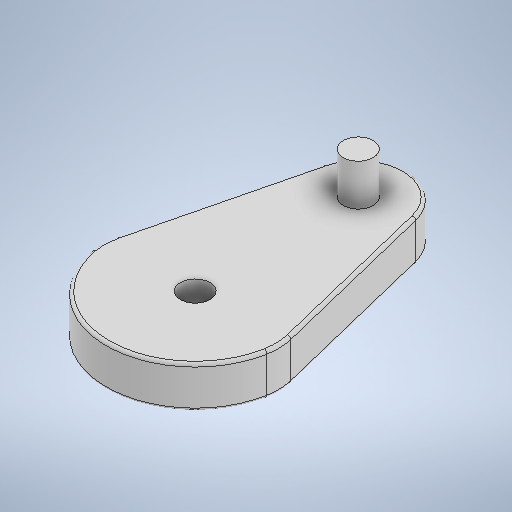
# Autodesk Inventor part: 202 part 1
Saved by Autodesk Inventor 2025.1 (Build 291241000, 241)
## iProperties
Created: 2024-09-02
Part Number: 202 part 1
Material: Generisch
Document SubType Name: Modeling
Designer: ffogue
Density: 1 g/cm^3
Appearance: Vorgabe
Author: ffogue
Autodesk Inventor part; units mm, degrees
ref_plane "YZ Plane" through (0, 0, 0) normal (1, 0, 0) x (0, 1, 0)
ref_plane "XZ Plane" through (0, 0, 0) normal (0, 1, 0) x (-1, 0, 0)
ref_plane "XY Plane" through (0, 0, 0) normal (0, 0, 1) x (1, 0, 0)
sketch "Sketch1" plane through (0, 0, 0) normal (0, 0, 1) x (1, 0, 0)
  line L0 (-15, 0) -> (15, 0) construction
  arc A0 (-15, 0) -> (15, 0) centre (0, 0) ccw
  line L1 (-15, 0) -> (-7.7686, 29.4102)
  arc A1 (7.7686, 29.4102) -> (-7.7686, 29.4102) centre (0, 27.5) ccw
  line L2 (7.7686, 29.4102) -> (15, 0)
  circle A2 centre (0, 0) radius 2.5
  circle A3 centre (0, 27.5) radius 2.5
  dimension "d0" = 8
  dimension "d1" = 15
  dimension "d2" = 27.5
  dimension "d3" = 5
  dimension "d10" = 5
  constraints: 6 end point, 4 centre point, 4 point on circle, 3 coincident, 2 horizontal alignment, 2 midpoint, 1 horizontal, 1 tangent, 1 vertical alignment
  measures "d0" radius of A1
  measures "d1" radius of A0
  measures "d2" distance of point (0, 0) A1.centre
  measures "d3" diameter of A2
  measures "d10" diameter of A3
extrude "Extrusion1" add sketch "Sketch1" against normal blind 7 contours L1 A1 L2 A0 | A3
fillet "Fillet1" radius 10 2 edges at (15, 0, -3.5) (-15, 0, -3.5)
fillet "Fillet2" radius 0.5 12 edges at (0, 35.5, 0) (-11.1999, 15.4549, 0) (-14.9156, -0.5754, 0) (0, -15, 0) (14.9156, -0.5754, 0) (11.1999, 15.4549, 0) (14.9156, -0.5754, -7) (0, -15, -7) (-14.9156, -0.5754, -7) (-11.1999, 15.4549, -7) (0, 35.5, -7) (11.1999, 15.4549, -7)
extrude "Extrusion2" add sketch "Sketch1" along normal blind 7 separate body contours A3
body "Solid1"
body "Solid2"
